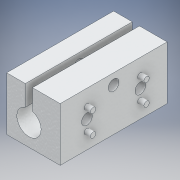
# Autodesk Inventor part: SupportV2_P1_ComFuros
Saved by Autodesk Inventor 2017 (Build 210142000, 142)
## iProperties
Created: 2023-04-27
Part Number: SupportV2_P1_ComFuros
Material: PET Plastic
Document SubType Name: Modeling
Designer: Vinicius Silva
Density: 1.541 g/cm^3
Appearance: White
Author: Vinicius Silva
Autodesk Inventor part; units mm, degrees
ref_plane "YZ Plane" through (0, 0, 0) normal (1, 0, 0) x (0, 1, 0)
ref_plane "XZ Plane" through (0, 0, 0) normal (0, 1, 0) x (-1, 0, 0)
ref_plane "XY Plane" through (0, 0, 0) normal (0, 0, 1) x (1, 0, 0)
sketch "Sketch1" plane through (0, 0, 0) normal (0, 1, 0) x (-1, 0, 0)
  line L0 (30, 0) -> (30, -30)
  line L1 (30, -30) -> (0, -30)
  line L2 (0, -30) -> (0, 0)
  arc A0 (15.5, -11.5008) -> (19.5, -11.5008) centre (17.5, -18) ccw
  line L3 (17.5, -18) -> (17.5, -3) construction
  line L4 (15.5, 0) -> (15.5, -11.5008)
  line L5 (19.5, -11.5008) -> (19.5, 0)
  line L6 (0, 0) -> (15.5, 0)
  line L7 (19.5, 0) -> (30, 0)
  dimension "d0" = 30
  dimension "d1" = 30
  dimension "d2" = 13.6
  dimension "d3" = 18
  dimension "d8" = 17.5
  dimension "d9" = 4
  dimension "d10" = 2
  constraints: 16 end point, 6 parallel, 2 horizontal, 2 perpendicular, 2 point on circle, 1 centre point, 1 coincident
  measures "d0" distance of L0.end L1.end
  measures "d1" distance of L0.start L0.end
  measures "d2" diameter of A0
  measures "d3" vertical distance of L2.end L3.start
  measures "d8" distance from line of L2 L3.start
  measures "d9" distance between parallel lines of L5 L4
  measures "d10" distance between parallel lines of L5 L3
extrude "Extrusion1" add sketch "Sketch1" along normal blind 60
sketch "Sketch2" plane through (0, 0, 0) normal (1, 0, 0) x (0, 0, -1)
  line L0 (0, 0) -> (30, 0) projected
  line L1 (30, 0) -> (30, 60) projected
  line L2 (0, 60) -> (30, 60) projected
  line L3 (0, 0) -> (0, 60) projected
  line L4 (11.5008, 0) -> (11.5008, 60) projected
  circle A0 centre (6, 30) radius 3
  dimension "d14" = 6
  dimension "d15" = 30
  dimension "d16" = 6
  constraints: 1 centre point
  measures "d14" diameter of A0
  measures "d15" distance from line of L0 A0.centre
  measures "d16" distance from line of L3 A0.centre
extrude "Extrusion2" cut sketch "Sketch2" against normal through all contours A0
sketch "Sketch3" plane through (-30, 0, -30) normal (-1, 0, 0) x (0, 0, 1)
  line L0 (30, 0) -> (30, 60) projected
  circle A0 centre (24, 30) radius 3 construction
  line L1 (19.7, 27.5174) -> (19.7, 32.4826)
  line L2 (19.7, 32.4826) -> (24, 34.9652)
  line L3 (24, 34.9652) -> (28.3, 32.4826)
  line L4 (28.3, 32.4826) -> (28.3, 27.5174)
  line L5 (28.3, 27.5174) -> (24, 25.0348)
  line L6 (24, 25.0348) -> (19.7, 27.5174)
  dimension "d31" = 4.3
  constraints: 12 end point, 1 coincident, 1 parallel, 13 other
  measures "d31" distance from line of point (24, 30) L4
sketch "Sketch4" plane through (0, 0, 0) normal (1, 0, 0) x (0, 0, -1)
  circle A0 centre (6, 30) radius 3 construction
  line L0 (0, 0) -> (30, 0) construction
  line L1 (30, 0) -> (30, 60) construction
  line L2 (0, 60) -> (30, 60) construction
  line L3 (0, 0) -> (0, 60) construction
  line L4 (30, 60) -> (0, 60) construction
  line L5 (15, 60) -> (15, 0) construction
  line L6 (30, 0) -> (0, 0) construction
  line L7 (0, 0) -> (0, 60) construction
  line L8 (0, 30) -> (30, 30) construction
  circle A1 centre (15, 45) radius 3
  circle A2 centre (15, 15) radius 3
  dimension "d22" = 6
  dimension "d23" = 15
  dimension "d24" = 6
  dimension "d25" = 15
  constraints: 4 end point, 4 midpoint, 2 centre point, 2 point on line
  measures "d22" diameter of A1
  measures "d23" distance from line of L2 A1.centre
  measures "d24" diameter of A2
  measures "d25" distance from line of L0 A2.centre
extrude "Extrusion4" cut sketch "Sketch4" against normal blind 10
extrude "Extrusion6" cut sketch "Sketch3" against normal blind 4
sketch "Sketch6" plane through (0, 0, 0) normal (1, 0, 0) x (0, 0, -1)
  circle A0 centre (15, 45) radius 3 construction
  circle A1 centre (15, 15) radius 3 construction
  circle A2 centre (6, 30) radius 3 construction
  line L0 (0, 0) -> (30, 0) construction
  line L1 (30, 0) -> (30, 60) construction
  line L2 (0, 60) -> (30, 60) construction
  line L3 (0, 0) -> (0, 60) construction
  line L4 (30, 0) -> (30, 60) construction
  line L5 (30, 15) -> (0, 15) construction
  line L6 (30, 45) -> (0, 45) construction
  line L7 (0, 0) -> (0, 60) construction
  circle A3 centre (9, 15) radius 1.5
  circle A4 centre (21, 15) radius 1.5
  circle A5 centre (9, 45) radius 1.5
  circle A6 centre (21, 45) radius 1.5
  dimension "d34" = 3
  dimension "d35" = 3
  dimension "d36" = 3
  dimension "d37" = 3
  dimension "d38" = 6
  dimension "d39" = 6
  dimension "d40" = 6
  dimension "d41" = 6
  dimension "d42" = 15
  dimension "d43" = 15
  constraints: 8 point on line, 4 centre point, 4 end point, 1 horizontal, 1 parallel
  measures "d34" diameter of A3
  measures "d35" diameter of A4
  measures "d36" diameter of A5
  measures "d37" diameter of A6
  measures "d38" distance of A1.centre A3.centre
  measures "d39" distance of A1.centre A4.centre
  measures "d40" distance of A0.centre A5.centre
  measures "d41" distance of A0.centre A6.centre
  measures "d42" distance between parallel lines of L0 L5
  measures "d43" distance between parallel lines of L2 L6
extrude "Extrusion7" add sketch "Sketch6" along normal blind 3.5
sketch "Sketch7" plane through (0, 60, 0) normal (0, 1, 0) x (1, 0, 0)
  circle A0 centre (-5.5, 24.5) radius 3
  line L0 (0, 30) -> (-30, 30) projected
  line L1 (0, 0) -> (0, 30) projected
  dimension "d46" = 6
  dimension "d47" = 5.5
  dimension "d48" = 5.5
  constraints: 1 centre point
  measures "d46" diameter of A0
  measures "d47" distance from line of L0 A0.centre
  measures "d48" distance from line of L1 A0.centre
extrude "Extrusion8" cut sketch "Sketch7" against normal blind 15
body "Solid1"
